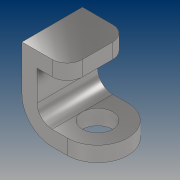
# Autodesk Inventor part: 18
Saved by Autodesk Inventor 2020.2 (Build 242310000, 310)
## iProperties
Created: 2020-09-17
Part Number: 18
Material: 鋼、碳鋼
Document SubType Name: Modeling
Designer: user
Density: 7.85 g/cm^3
Appearance: 半拋光
Mass: 283.677 g
Surface Area: 104.695 cm^2
Volume: 36.1372 cm^3
Author: user
Autodesk Inventor part; units mm, degrees
ref_plane "YZ Plane" through (0, 0, 0) normal (1, 0, 0) x (0, 1, 0)
ref_plane "XZ Plane" through (0, 0, 0) normal (0, 1, 0) x (-1, 0, 0)
ref_plane "XY Plane" through (0, 0, 0) normal (0, 0, 1) x (1, 0, 0)
sketch "草圖1" plane through (0, 0, 0) normal (0, 0, 1) x (1, 0, 0)
  line L0 (0, 0) -> (-30, 0)
  line L1 (-30, 0) -> (-30, -30)
  arc A0 (-30, -30) -> (-10, -50) centre (-10, -30) ccw
  line L2 (-10, -50) -> (20, -50)
  line L3 (20, -50) -> (20, -40)
  line L4 (20, -40) -> (-10, -40)
  arc A1 (-20, -30) -> (-10, -40) centre (-10, -30) ccw
  line L5 (-20, -30) -> (-20, -10)
  line L6 (-20, -10) -> (0, -10)
  line L7 (0, -10) -> (0, 0)
  dimension "d0" = 10
  dimension "d1" = 50
  dimension "d2" = 10
  dimension "d3" = 20
  dimension "d4" = 30
  dimension "d5" = 10
  constraints: 16 end point, 7 perpendicular, 4 point on circle, 4 tangent, 2 centre point, 1 concentric, 1 horizontal
  measures "d0" distance of L6.end L0.start
  measures "d1" distance between parallel lines of L0 L2
  measures "d2" distance of L2.end L3.end
  measures "d3" distance between parallel lines of L3 L7
  measures "d4" distance of L0.start L0.end
  measures "d5" radius of A1
extrude "擠出1" add sketch "草圖1" along normal mid plane 40
fillet "圓角1" radius 10 2 edges at (0, -5, 20) (0, -5, -20)
fillet "圓角2" radius 20 2 edges at (20, -45, 20) (20, -45, -20)
sketch "草圖2" plane through (-10, -40, 20) normal (0, 1, 0) x (1, 0, 0)
  arc A0 (10, 0) -> (10, 40) centre (10, 20) ccw projected
  point P0 (10, 20)
  constraints: 1 coincident
hole "孔1" at (0, -40, 0) direction (0, -1, 0) diameter 20 end through all
